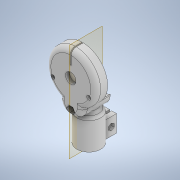
# Autodesk Inventor part: Motorconnection
Saved by Autodesk Inventor 2021 (Build 250183000, 183)
## iProperties
Created: 2021-03-16
Part Number: Motorconnection
Material: Generic
Document SubType Name: Modeling
Designer: Olivi
Density: 1 g/cm^3
Appearance: Default
Author: Olivi
Autodesk Inventor part; units mm, degrees
ref_plane "YZ Plane" through (0, 0, 0) normal (1, 0, 0) x (0, 1, 0)
ref_plane "XZ Plane" through (0, 0, 0) normal (0, 1, 0) x (-1, 0, 0)
ref_plane "XY Plane" through (0, 0, 0) normal (0, 0, 1) x (1, 0, 0)
sketch "Sketch1" plane through (0, 0, 0) normal (0, 0, 1) x (1, 0, 0)
  circle A0 centre (0, 0) radius 25
  dimension "d0" = 50
  constraints: 1 centre point, 1 coincident
  measures "d0" diameter of A0
extrude "Extrusion1" add sketch "Sketch1" along normal blind 12
sketch "Sketch2" plane through (0, 0, 12) normal (0, 0, 1) x (1, 0, 0)
  line L0 (6.4, -24) -> (6.4, -19.8844) construction
  line L1 (6.4, -19.8844) -> (7.4, -19.8844) construction
  arc A0 (7.4, -19.8844) -> (13.6748, -11) centre (0, -8) ccw construction
  line L2 (13.6748, -11) -> (18, -11) construction
  arc A1 (18, -11) -> (18, -5) centre (18, -8) ccw construction
  line L3 (18, -5) -> (13.6748, -5) construction
  arc A2 (13.6748, -5) -> (-13.6748, -5) centre (0, -8) ccw construction
  line L4 (-13.6748, -5) -> (-18, -5) construction
  arc A3 (-18, -5) -> (-18, -11) centre (-18, -8) ccw construction
  line L5 (-18, -11) -> (-13.6748, -11) construction
  arc A4 (-13.6748, -11) -> (-7.4, -19.8844) centre (0, -8) ccw construction
  line L6 (-7.4, -19.8844) -> (-6.4, -19.8844) construction
  line L7 (-6.4, -19.8844) -> (-6.4, -24) construction
  line L8 (-6.4, -24) -> (6.4, -24) construction
  line L9 (8.75, -20.0582) -> (8.75, -18.9287) construction
  arc A5 (7.4, -19.8844) -> (8.75, -18.9287) centre (0, -8) ccw construction
  line L10 (7.4, -19.8844) -> (7.4, -22) construction
  line L11 (7.4, -22) -> (8.5085, -20.7098) construction
  arc A6 (8.5085, -20.7098) -> (8.75, -20.0582) centre (7.75, -20.0582) ccw construction
  arc A7 (-8.75, -18.9287) -> (-7.4, -19.8844) centre (0, -8) ccw construction
  line L12 (-8.75, -18.9287) -> (-8.75, -20.0582) construction
  arc A8 (-8.75, -20.0582) -> (-8.5085, -20.7098) centre (-7.75, -20.0582) ccw construction
  line L13 (-8.5085, -20.7098) -> (-7.4, -22) construction
  line L14 (-7.4, -22) -> (-7.4, -19.8844) construction
  line L15 (7.4, -19.8844) -> (6.4, -19.8844) construction
  line L16 (6.4, -19.8844) -> (6.4, -24) construction
  line L17 (6.4, -24) -> (-6.4, -24) construction
  line L18 (-6.4, -24) -> (-6.4, -19.8844) construction
  line L19 (-6.4, -19.8844) -> (-7.4, -19.8844) construction
  arc A9 (7.4, -19.8844) -> (13.6748, -11) centre (0, -8) ccw construction
  line L20 (13.6748, -11) -> (18, -11) construction
  arc A10 (18, -11) -> (18, -5) centre (18, -8) ccw construction
  line L21 (18, -5) -> (13.6748, -5) construction
  arc A11 (13.6748, -5) -> (-13.6748, -5) centre (0, -8) ccw construction
  line L22 (-13.6748, -5) -> (-18, -5) construction
  arc A12 (-18, -5) -> (-18, -11) centre (-18, -8) ccw construction
  line L23 (-18, -11) -> (-13.6748, -11) construction
  arc A13 (-13.6748, -11) -> (-7.4, -19.8844) centre (0, -8) ccw construction
  line L24 (-7.4, -19.8844) -> (-7.4, -24) construction
  arc A14 (-7.4, -24) -> (-6.4, -25) centre (-6.4, -24) ccw construction
  line L25 (-6.4, -25) -> (6.4, -25) construction
  arc A15 (6.4, -25) -> (7.4, -24) centre (6.4, -24) ccw construction
  line L26 (7.4, -24) -> (7.4, -19.8844) construction
  circle A16 centre (0, 0) radius 4.5 construction
  circle A17 centre (18, -8) radius 2 construction
  circle A18 centre (-18, -8) radius 2 construction
  circle A19 centre (0, 0) radius 0.75 construction
  line L27 (8.5085, -20.7098) -> (7.4, -22) construction
  arc A20 (1.5, -22.4222) -> (8.75, -19.5623) centre (0, -8) ccw construction
  circle A21 centre (-18, -8) radius 2
  circle A22 centre (18, -8) radius 2
  point P0 (0, 0)
  constraints: 56 end point, 38 point on circle, 23 centre point, 3 point on line, 2 coincident, 2 concentric
extrude "Extrusion2" cut sketch "Sketch2" against normal through all
sketch "Sketch3" plane through (0, 0, 12) normal (0, 0, 1) x (1, 0, 0)
  circle A0 centre (0, 0) radius 5.25
  dimension "d5" = 10.5
  constraints: 1 centre point, 1 coincident
  measures "d5" diameter of A0
extrude "Extrusion3" cut sketch "Sketch3" against normal through all
sketch "Sketch4" plane through (0, 0, 0) normal (0, 0, -1) x (-1, 0, 0)
  circle A0 centre (0, 0) radius 11.25
  dimension "d8" = 22.5
  constraints: 1 centre point, 1 coincident
  measures "d8" diameter of A0
extrude "Extrusion4" cut sketch "Sketch4" against normal blind 8
sketch "Sketch5" plane through (0, 0, 0) normal (0, 0, -1) x (-1, 0, 0)
  circle A0 centre (-18, -8) radius 2 projected
  line L0 (-14.5359, -8) -> (-16.2679, -11)
  line L1 (-16.2679, -11) -> (-19.7321, -11)
  line L2 (-19.7321, -11) -> (-21.4641, -8)
  line L3 (-21.4641, -8) -> (-19.7321, -5)
  line L4 (-19.7321, -5) -> (-16.2679, -5)
  line L5 (-16.2679, -5) -> (-14.5359, -8)
  circle A1 centre (18, -8) radius 2 projected
  line L6 (19.7719, -11) -> (16.2879, -11.0345)
  line L7 (16.2879, -11.0345) -> (14.516, -8.0345)
  line L8 (14.516, -8.0345) -> (16.2281, -5)
  line L9 (16.2281, -5) -> (19.7121, -4.9655)
  line L10 (19.7121, -4.9655) -> (21.484, -7.9655)
  line L11 (21.484, -7.9655) -> (19.7719, -11)
  point P0 (0, 0)
  dimension "d11" = 6
  constraints: 24 end point, 2 coincident, 26 other
  measures "d11" distance between parallel lines of L1 L4
extrude "Extrusion5" cut sketch "Sketch5" against normal blind 8 contours A0 | L0 L1 L2 L3 L4 L5 | A1 | L6 L7 L8 L9 L10 L11
sketch "Sketch6" plane through (0, 0, 12) normal (0, 0, 1) x (1, 0, 0)
  line L0 (-11.5, -16.5) -> (11.5, -16.5)
  line L1 (11.5, -16.5) -> (11.5, -33.5)
  line L2 (11.5, -33.5) -> (-11.5, -33.5)
  line L3 (-11.5, -33.5) -> (-11.5, -16.5)
  circle A0 centre (0, 0) radius 25 projected
  line L4 (-11.5, -16.5) -> (11.5, -33.5) construction
  line L5 (11.5, -16.5) -> (-11.5, -33.5) construction
  arc A1 (-11.5, -22.198) -> (11.5, -22.198) centre (0, 0) ccw
  point P0 (0, -25)
  dimension "d14" = 23
  dimension "d18" = 17
  constraints: 12 end point, 6 point on circle, 2 midpoint, 2 parallel, 2 point on line, 1 centre point, 1 horizontal, 1 perpendicular
  measures "d14" distance of L1.end L2.end
  measures "d18" distance of L0.end L1.end
extrude "Extrusion6" add sketch "Sketch6" against normal blind 28 contours A0 L1 L2 L3
fillet "Fillet1" radius 10 2 edges at (-11.5, -33.5, -2) (11.5, -33.5, -2)
sketch "Sketch7" plane through (0, 0, -16) normal (0, 0, -1) x (-1, 0, 0)
  circle A0 centre (0.0022, -28) radius 2.25
  line L0 (-1.5, -33.5) -> (1.5, -33.5) projected
  point P0 (0, 0)
  dimension "d19" = 4.5
  dimension "d20" = 5.5
  constraints: 1 centre point
  measures "d19" diameter of A0
  measures "d20" distance from line of L0 A0.centre
extrude "Extrusion7" cut sketch "Sketch7" against normal through all
sketch "Sketch8" plane through (0, 0, 12) normal (0, 0, 1) x (1, 0, 0)
  circle A0 centre (-0.0022, -28) radius 2.25 projected
  line L0 (-4.2168, -28) -> (-2.1095, -24.35)
  line L1 (-2.1095, -24.35) -> (2.1052, -24.35)
  line L2 (2.1052, -24.35) -> (4.2125, -28)
  line L3 (4.2125, -28) -> (2.1052, -31.65)
  line L4 (2.1052, -31.65) -> (-2.1095, -31.65)
  line L5 (-2.1095, -31.65) -> (-4.2168, -28)
  point P0 (0, 0)
  dimension "d23" = 7.3
  constraints: 12 end point, 1 coincident, 13 other
  measures "d23" distance between parallel lines of L1 L4
extrude "Extrusion8" cut sketch "Sketch8" against normal blind 5 contours A0 | L0 L1 L2 L3 L4 L5
fillet "Fillet2" radius 5 6 edges at (0, 25, 12) (-11.5, -22.849, 12) (0, -33.5, 12) (8.5711, -30.5711, 12) (11.5, -22.849, 12) (-8.5711, -30.5711, 12)
sketch "Sketch10" plane through (-1.5, -33.5, -16) normal (0, -1, 0) x (1, 0, 0)
  point P0 (1.5, 16)
sketch "Sketch12" plane through (-1.5, -33.5, -16) normal (0, -1, 0) x (1, 0, 0)
  circle A0 centre (1.5, 9.883) radius 8
  line L0 (3, 26.883) -> (0, 26.883) projected
  point P0 (1.5, 16)
  dimension "d31" = 16
  dimension "d32" = 17
  constraints: 1 centre point
  measures "d31" diameter of A0
  measures "d32" distance from line of L0 A0.centre
extrude "Extrusion10" add sketch "Sketch12" along normal mid plane 3
sketch "Sketch13" plane through (0, -35, -6.117) normal (0, -1, 0) x (1, 0, 0)
  circle A0 centre (0, 0) radius 7.75
  circle A1 centre (0, 0) radius 12
  point P0 (0, 6.117)
  dimension "d35" = 15.5
  dimension "d36" = 24
  constraints: 2 centre point, 1 coincident
  measures "d35" diameter of A0
  measures "d36" diameter of A1
extrude "Extrusion11" add sketch "Sketch13" along normal blind 30
fillet "Fillet3" radius 3 1 edges at (-8, -35, -6.117)
fillet "Fillet4" radius 3 1 edges at (-12, -35, -6.117)
sketch "Sketch14" plane through (0, -65, -6.117) normal (0, -1, 0) x (1, 0, 0)
  point P0 (0, 6.117)
ref_plane "Work Plane3" through (0, -22.198, 0) normal (1, 0, 0) x (0, 0, -1)
sketch "Sketch16" plane through (0, -22.198, 0) normal (1, 0, 0) x (0, 0, -1)
  line L0 (-5.883, -42.802) -> (18.117, -42.802) projected
  line L1 (18.117, -42.802) -> (12.4039, -42.802)
  line L2 (12.4039, -42.802) -> (12.4039, -12.6305)
  line L3 (-3.883, -12.6305) -> (16.117, -12.6305) projected
  line L4 (12.4039, -12.6305) -> (18.117, -12.6305)
  line L5 (18.117, -12.6305) -> (18.117, -42.802)
  point P0 (0, 22.198)
  constraints: 8 end point, 2 perpendicular, 2 point on line, 1 horizontal
extrude "Extrusion13" cut sketch "Sketch16" along normal mid plane 2
sketch "Sketch17" plane through (0, -65, -6.117) normal (0, -1, 0) x (1, 0, 0)
  arc A0 (1, -11.9583) -> (-1, -11.9583) centre (0, 0) ccw projected
  line L0 (1, -11.9583) -> (1, -22.0279)
  line L1 (1, -22.0279) -> (5.8364, -22.0279)
  line L2 (5.8364, -22.0279) -> (5.8364, -10.485)
  line L3 (-1, -11.9583) -> (-1, -22.0279)
  line L4 (-1, -22.0279) -> (-6.0626, -22.0279)
  line L5 (-6.0626, -22.0279) -> (-6.0626, -10.3559)
  arc A1 (1, -11.9583) -> (5.8364, -10.485) centre (0, 0) ccw
  arc A2 (-6.0626, -10.3559) -> (-1, -11.9583) centre (0, 0) ccw
  point P0 (0, 6.117)
  constraints: 12 end point, 6 point on circle, 3 concentric, 3 perpendicular, 2 centre point, 2 point on line, 1 parallel, 1 vertical
extrude "Extrusion14" add sketch "Sketch17" against normal blind 17
sketch "Sketch18" plane through (-6.0626, -65, -28.1449) normal (-1, 0, 0) x (0, 0, 1)
  circle A0 centre (5.2721, 8.0429) radius 1.75
  point P0 (28.1449, 65)
  dimension "d49" = 3.5
  constraints: 1 centre point
  measures "d49" diameter of A0
extrude "Extrusion15" cut sketch "Sketch18" against normal blind 17
sketch "Sketch19" plane through (-6.0626, -65, -28.1449) normal (-1, 0, 0) x (0, 0, 1)
  circle A0 centre (5.2721, 8.0429) radius 1.75 projected
  circle A1 centre (5.2721, 8.0429) radius 3
  point P0 (28.1449, 65)
  dimension "d52" = 6
  constraints: 1 centre point, 1 coincident
  measures "d52" diameter of A1
extrude "Extrusion16" cut sketch "Sketch19" against normal blind 2.5 contours A0 | A1
sketch "Sketch20" plane through (5.8364, -65, -16.6021) normal (1, 0, 0) x (0, 0, -1)
  circle A0 centre (6.2708, 8.0429) radius 1.75 projected
  line L0 (6.2708, 4.752) -> (3.4208, 6.3974)
  line L1 (3.4208, 6.3974) -> (3.4208, 9.6883)
  line L2 (3.4208, 9.6883) -> (6.2708, 11.3338)
  line L3 (6.2708, 11.3338) -> (9.1208, 9.6883)
  line L4 (9.1208, 9.6883) -> (9.1208, 6.3974)
  line L5 (9.1208, 6.3974) -> (6.2708, 4.752)
  point P0 (-16.6021, 65)
  dimension "d55" = 5.7
  constraints: 12 end point, 1 coincident, 13 other
  measures "d55" distance between parallel lines of L1 L4
extrude "Extrusion17" cut sketch "Sketch20" against normal blind 2.5 contours A0 | L0 L1 L2 L3 L4 L5
sketch "Sketch21" plane through (0, 0, 0) normal (0, 0, -1) x (-1, 0, 0)
  circle A0 centre (0, 0) radius 11.25 projected
  line L0 (0, 11.25) -> (0.4999, 11.2389)
  line L1 (0, 11.25) -> (0, 26.6648)
  line L2 (0, 26.6648) -> (0.4999, 26.6648)
  line L3 (0.4999, 26.6648) -> (0.4999, 11.2389)
  line L4 (0, 11.25) -> (0, 26.6648)
  line L5 (0, 26.6648) -> (-0.5, 26.6648)
  line L6 (-0.5, 26.6648) -> (-0.5, 11.2389)
  dimension "d58" = 0.5
  dimension "d59" = 0.5
  constraints: 14 end point, 3 perpendicular, 3 point on circle, 1 parallel, 1 point on line, 1 vertical
  measures "d58" distance of L0.start L0.end
  measures "d59" distance of L1.end L5.end
extrude "Extrusion18" cut sketch "Sketch21" against normal through all contours A0 L1 L2 L3 | L6 L5 L1 A0
fillet "Fillet5" radius 5 1 edges at (0, -35, 1.633)
body "Solid1"
